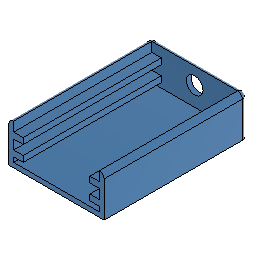
Base Station Enclosure - V15 (Autodesk Fusion 360 design; units mm, degrees)
Autodesk Fusion 360 part; units mm, degrees
sketch "Sketch1" plane through (0, 0, 0) normal (0, 0, 1) x (1, 0, 0)
  line L0 (0, 0) -> (40, 0)
  line L1 (40, 0) -> (40, 60)
  line L2 (40, 60) -> (0, 60)
  line L3 (0, 60) -> (0, 0)
  line L4 (0, 60) -> (2, 60)
  line L5 (2, 60) -> (2, 58)
  line L6 (40, 0) -> (38, 0)
  line L7 (38, 0) -> (38, 2)
  line L8 (2, 58) -> (38, 58)
  line L9 (38, 58) -> (38, 2)
  line L10 (38, 2) -> (2, 2)
  line L11 (2, 2) -> (2, 58)
  line L12 (0, 60) -> (-10, 60)
  line L13 (-10, 60) -> (-10, 45)
  line L14 (-10, 45) -> (0, 45)
  line L15 (20, 60) -> (20, 87)
  line L16 (50, 60) -> (50, 45)
  line L17 (50, 45) -> (40, 45)
  line L18 (40, 60) -> (50, 60)
  line L19 (-10, 60) -> (-7, 60)
  line L20 (0, 60) -> (-2, 60)
  line L21 (-2, 60) -> (-2, 45)
  line L22 (-10, 45) -> (-7, 45)
  line L23 (-7, 45) -> (-7, 48)
  line L24 (-7, 48) -> (-2, 48)
  line L25 (-7, 60) -> (-7, 57)
  line L26 (-7, 57) -> (-2, 57)
  line L27 (-7, 57) -> (-7, 48)
  line L28 (-2, 57) -> (0, 57)
  line L29 (-2, 48) -> (0, 48)
  dimension "d1" = 40
  dimension "d2" = 60
  dimension "d3" = 2
  dimension "d4" = 2
  dimension "d5" = 2
  dimension "d6" = 2
  dimension "d40" = 10
  dimension "d41" = 15
  dimension "d60" = 3
  dimension "d61" = 2
  dimension "d62" = 3
  dimension "d63" = 3
  dimension "d64" = 3
  constraint horizontal L0
  constraint vertical L1
  constraint horizontal L2
  constraint vertical L3
  constraint coincident L0.start L3.end
  constraint perpendicular L3 L4
  constraint perpendicular L2 L5
  constraint perpendicular L1 L6
  constraint perpendicular L6 L7
  constraint horizontal L8
  constraint vertical L9
  constraint horizontal L10
  constraint vertical L11
  constraint perpendicular L3 L12
  constraint perpendicular L2 L13
  constraint coincident L3 L14.end
  constraint perpendicular L3 L14
  constraint midpoint L2 L15.start
  constraint perpendicular L2 L15
  constraint symmetric L2.end L15 L1.end
  constraint symmetric L12.end L15 L16.start
  constraint symmetric L13.end L15 L16.end
  constraint symmetric L14.end L15 L17.end
  constraint coincident L12 L19.end
  constraint perpendicular L3 L20
  constraint coincident L14 L21.end
  constraint perpendicular L14 L21
  constraint perpendicular L13 L22
  constraint perpendicular L22 L23
  constraint coincident L21 L24.end
  constraint perpendicular L21 L24
  constraint perpendicular L19 L25
  constraint coincident L21 L26.end
  constraint perpendicular L21 L26
  constraint coincident L3 L28.end
  constraint perpendicular L3 L28
  constraint coincident L3 L29.end
  constraint perpendicular L3 L29
  measures "d1" distance of L0.start L0.end
  measures "d2" distance of L0.start L2.end
  measures "d3" distance of L2.end L4.end
  measures "d4" distance of L4.end L5.end
  measures "d5" distance of L0.end L6.end
  measures "d6" distance of L6.end L7.end
  measures "d40" distance of L2.end L12.end
  measures "d41" distance of L12.end L13.end
  measures "d60" distance of L12.end L19.end
  measures "d61" distance of L2.end L20.end
  measures "d62" distance of L13.end L22.end
  measures "d63" distance of L22.end L23.end
  measures "d64" distance of L19.end L25.end
extrude "Extrude1" add sketch "Sketch1" along normal blind 2 contours L8 L9 L10 L11
extrude "Extrude2" add sketch "Sketch1" along normal blind 25 contours L0 L2 L3 L4 L5 L7 L10 L11 | L0 L1 L2 L5 L6 L7 L8 L9
sketch "Sketch6" plane through (0, 0, 25) normal (0, 0, 1) x (-1, 0, 0)
  line L0 (-38, -2) -> (-2, -2)
  line L1 (-2, -2) -> (-2, -58)
  line L2 (-2, -58) -> (-38, -58)
  line L3 (-38, -58) -> (-38, -2)
  line L4 (-40, -60) -> (0, -60)
  line L5 (0, -60) -> (0, 0)
  line L6 (0, 0) -> (-40, 0)
  line L7 (-40, 0) -> (-40, -60)
  line L8 (-38, -2) -> (-38, 0)
  line L9 (-2, -2) -> (-2, 0)
  constraint coincident L0.start L3.end
  constraint coincident L6 L8.end
  constraint perpendicular L6 L8
  constraint coincident L0.end L1.start
  constraint coincident L6 L9.end
  constraint perpendicular L0 L9
extrude "Extrude10" cut sketch "Sketch6" against normal blind 23 contours L0 L6 L8 L9
sketch "Sketch7" plane through (0, 0, 0) normal (0, -1, 0) x (1, 0, 0)
  line L0 (2, 2) -> (2, 25)
  line L1 (2, 25) -> (0, 25)
  line L2 (0, 25) -> (0, 0)
  line L3 (0, 0) -> (40, 0)
  line L4 (40, 0) -> (40, 25)
  line L5 (40, 25) -> (38, 25)
  line L6 (38, 25) -> (38, 2)
  line L7 (38, 2) -> (2, 2)
  line L8 (2, 2) -> (2, 4)
  line L9 (2, 4) -> (6, 4)
  line L10 (6, 4) -> (6, 6.5)
  line L11 (6, 6.5) -> (2, 6.5)
  line L12 (2, 25) -> (2, 13)
  line L13 (2, 13) -> (6, 13)
  line L14 (6, 13) -> (6, 10.5)
  line L15 (6, 10.5) -> (2, 10.5)
  line L16 (20, 0) -> (20, -5)
  line L17 (38, 4) -> (34, 4)
  line L18 (34, 4) -> (34, 6.5)
  line L19 (34, 6.5) -> (38, 6.5)
  line L20 (34, 10.5) -> (38, 10.5)
  line L21 (34, 13) -> (34, 10.5)
  line L22 (38, 13) -> (34, 13)
  dimension "d75" = 2
  dimension "d76" = 4
  dimension "d77" = 2.5
  dimension "d78" = 12
  dimension "d79" = 4
  dimension "d80" = 2.5
  constraint coincident L0.start L7.end
  constraint perpendicular L7 L8
  constraint perpendicular L8 L9
  constraint perpendicular L9 L10
  constraint coincident L0 L11.end
  constraint perpendicular L0 L11
  constraint coincident L0.end L1.start
  constraint coincident L0 L12.end
  constraint perpendicular L12 L13
  constraint perpendicular L13 L14
  constraint coincident L0 L15.end
  constraint perpendicular L0 L15
  constraint midpoint L3 L16.start
  constraint perpendicular L3 L16
  constraint symmetric L8.end L16 L17.start
  constraint symmetric L9.end L16 L17.end
  constraint symmetric L10.end L16 L18.end
  constraint symmetric L11.end L16 L19.end
  constraint symmetric L12.end L16 L22.start
  constraint symmetric L13.end L16 L21.start
  constraint symmetric L14.end L16 L20.start
  constraint symmetric L15.end L16 L20.end
  measures "d75" distance of L0.start L8.end
  measures "d76" distance of L8.end L9.end
  measures "d77" distance of L9.end L10.end
  measures "d78" distance of L0.end L12.end
  measures "d79" distance of L12.end L13.end
  measures "d80" distance of L13.end L14.end
extrude "Extrude11" add sketch "Sketch7" against normal blind 58 contours L0 L9 L10 L11 | L6 L17 L18 L19 | L0 L13 L14 L15 | L6 L20 L21 L22
sketch "Sketch8" plane through (0, 0, 0) normal (0, -1, 0) x (1, 0, 0)
  line L0 (0, 25) -> (0, 0)
  line L1 (0, 0) -> (40, 0)
  line L2 (40, 0) -> (40, 25)
  line L3 (38, 25) -> (38, 13)
  line L4 (38, 13) -> (34, 13)
  line L5 (34, 13) -> (34, 10.5)
  line L6 (34, 10.5) -> (38, 10.5)
  line L7 (38, 10.5) -> (38, 6.5)
  line L8 (38, 6.5) -> (34, 6.5)
  line L9 (34, 6.5) -> (34, 4)
  line L10 (34, 4) -> (38, 4)
  line L11 (38, 4) -> (38, 2)
  line L12 (38, 2) -> (2, 2)
  line L13 (2, 2) -> (2, 4)
  line L14 (2, 4) -> (6, 4)
  line L15 (6, 4) -> (6, 6.5)
  line L16 (6, 6.5) -> (2, 6.5)
  line L17 (2, 6.5) -> (2, 10.5)
  line L18 (2, 10.5) -> (6, 10.5)
  line L19 (6, 10.5) -> (6, 13)
  line L20 (6, 13) -> (2, 13)
  line L21 (2, 13) -> (2, 25)
  line L22 (0, 0) -> (0, 17)
  line L23 (0, 17) -> (40, 17)
  line L24 (0, 17) -> (49.5328, 17)
  line L25 (49.5328, 17) -> (49.5328, 30.8118)
  line L26 (49.5328, 30.8118) -> (0, 30.8118)
  line L27 (0, 30.8118) -> (0, 17)
  line L28 (2, 25) -> (0, 25)
  line L29 (40, 25) -> (38, 25)
  dimension "d87" = 17
  constraint coincident L0.end L1.start
  constraint perpendicular L1 L22
  constraint coincident L2 L23.end
  constraint perpendicular L2 L23
  constraint horizontal L24
  constraint vertical L25
  constraint horizontal L26
  constraint vertical L27
  measures "d87" distance of L0.end L22.end
extrude "Extrude13" cut sketch "Sketch8" against normal blind 78 contours L0 L21 L23 L24 L27 L28 | L2 L3 L21 L23 L24 L25 L26 L27 L28 L29 | L2 L3 L23 L24 L29
fillet "Fillet13" radius 2 2 edges at (0, 30, 17) (40, 30, 17)
sketch "Sketch9" plane through (0, 60, 0) normal (0, 1, 0) x (-1, 0, 0)
  arc A0 (-38, 17) -> (-40, 15) centre (-38, 15) ccw
  line L0 (-40, 15) -> (-40, 0)
  line L1 (-40, 0) -> (0, 0)
  line L2 (0, 0) -> (0, 15)
  arc A1 (0, 15) -> (-2, 17) centre (-2, 15) ccw
  line L3 (-2, 17) -> (-38, 17)
  line L4 (-20, 0) -> (-20, 10)
  circle A2 centre (-20, 10) radius 3.5
  dimension "d92" = 10
  dimension "d93" = 7
  constraint midpoint L1 L4.start
  constraint perpendicular L1 L4
  constraint coincident L4.end A2.centre
  measures "d92" distance of L4.start L4.end
  measures "d93" diameter of A2
extrude "Extrude14" cut sketch "Sketch9" against normal blind 2 contours A2
fillet "Fillet14" radius 2 5 edges at (40, 60, 7.5) (39.4142, 60, 16.4142) (20, 60, 17) (0.5858, 60, 16.4142) (0, 60, 7.5)
